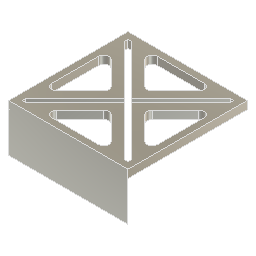
Нахождение центра для плоской турбы максимум до 40мм (Autodesk Fusion 360 design; units mm, degrees)
Autodesk Fusion 360 part; units mm, degrees
sketch "Sketch1" plane through (0, 0, 0) normal (0, 0, 1) x (1, 0, 0)
  line L0 (22.5, 22.5) -> (-22.5, 22.5)
  line L1 (-20, 20) -> (-20, 10)
  line L2 (22.5, -22.5) -> (22.5, 22.5)
  line L3 (20, -20) -> (10, -20)
  line L4 (-22.5, 22.5) -> (-22.5, -22.5)
  line L5 (-20, -20) -> (10, -20)
  line L6 (-20, 20) -> (-22.5, 22.5)
  line L7 (20, -20) -> (20, 20)
  line L8 (20, -20) -> (22.5, -22.5)
  line L9 (-20, 10) -> (-20, -20)
  line L10 (20, 20) -> (-20, 20)
  line L11 (-22.5, -22.5) -> (22.5, -22.5)
  line L12 (-18.5858, -20) -> (0, -1.4142)
  line L13 (1.4142, 0) -> (20, 18.5858)
  line L14 (18.5858, -20) -> (0, -1.4142)
  line L15 (-1.4142, 0) -> (-20, 18.5858)
  line L16 (-20, -18.5858) -> (-1.4142, 0)
  line L17 (0, 1.4142) -> (18.5858, 20)
  line L18 (20, -18.5858) -> (1.4142, 0)
  line L19 (0, 1.4142) -> (-18.5858, 20)
  line L20 (-18.5858, -20) -> (0, -1.4142)
  line L21 (1.4142, 0) -> (20, 18.5858)
  line L22 (-20, -18.5858) -> (-1.4142, 0)
  line L23 (0, 1.4142) -> (18.5858, 20)
  line L24 (20, -13.636) -> (6.364, 0)
  line L25 (0, 6.364) -> (-13.636, 20)
  line L26 (-20, -13.636) -> (-6.364, 0)
  line L27 (0, 6.364) -> (13.636, 20)
  line L28 (13.636, -20) -> (0, -6.364)
  line L29 (-6.364, 0) -> (-20, 13.636)
  line L30 (-20, -13.636) -> (-6.364, 0)
  line L31 (0, 6.364) -> (13.636, 20)
  line L32 (-13.636, -20) -> (0, -6.364)
  line L33 (6.364, 0) -> (20, 13.636)
  line L34 (6.364, 0) -> (20, 13.636)
  line L35 (-13.636, -20) -> (0, -6.364)
  line L36 (-20, -20) -> (-22.5, -22.5)
  line L37 (20, 20) -> (22.5, 22.5)
  dimension "d3" = 45
  dimension "d4" = 45
  constraint horizontal L5
  constraint perpendicular L5 L7
  constraint parallel L5 L10
  constraint parallel L7 L9
  constraint horizontal L11
  constraint perpendicular L2 L11
  constraint parallel L0 L11
  constraint parallel L2 L4
  constraint parallel L6 L8
  constraint coincident L32.start L5
  constraint coincident L26.start L9
  constraint coincident L3.start L5
  constraint coincident L1.start L9
  constraint coincident L5 L12.start
  constraint coincident L9 L16.start
  constraint coincident L7 L13.end
  constraint coincident L10 L17.end
  constraint coincident L10 L27.end
  constraint coincident L7 L33.end
  constraint collinear L12 L13
  constraint collinear L14 L15
  constraint coincident L17.start L18
  constraint collinear L16 L17
  constraint collinear L18 L19
  constraint collinear L20 L21
  constraint collinear L22 L23
  constraint collinear L24 L25
  constraint collinear L26 L27
  constraint collinear L28 L29
  constraint collinear L30 L31
  constraint collinear L32 L33
  constraint coincident L24.end L35
  constraint collinear L34 L35
  constraint parallel L36 L37
  measures "d3" distance of L0.start L0.end
  measures "d4" distance of L0.start L2.start
extrude "Extrude1" add sketch "Sketch1" along normal blind 3 contours L0 L6 L10 L37 | L2 L7 L8 L37 | L1 L4 L6 L9 L36 | L3 L5 L8 L11 L36 | L7 L13 L18 L21 L24 L33 L34 | L10 L17 L19 L23 L25 L27 L31 | L1 L9 L15 L16 L22 L26 L29 L30 | L3 L5 L12 L14 L20 L28 L32 L35
fillet "Fillet1" radius 2 12 edges at (-20, 13.636, 1.5) (-20, -13.636, 1.5) (-6.364, 0, 1.5) (0, -6.364, 1.5) (20, 13.636, 1.5) (-13.636, -20, 1.5) (6.364, 0, 1.5) (0, 6.364, 1.5) (13.636, -20, 1.5) (20, -13.636, 1.5) (13.636, 20, 1.5) (-13.636, 20, 1.5)
extrude "Extrude2" add sketch "Sketch1" against normal blind 15 contours L3 L5 L8 L11 L36
